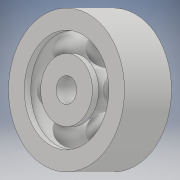
# Autodesk Inventor part: Подшипник
Saved by Autodesk Inventor 2018.1 (Build 221171000, 171)
## iProperties
Part Number: Подшипник
Material: Типовые
Document SubType Name: Modeling
Designer: User
Density: 1 g/cm^3
Appearance: По умолчанию
Author: User
Autodesk Inventor part; units mm, degrees
ref_plane "YZ Plane" through (0, 0, 0) normal (1, 0, 0) x (0, 1, 0)
ref_plane "XZ Plane" through (0, 0, 0) normal (0, 1, 0) x (-1, 0, 0)
ref_plane "XY Plane" through (0, 0, 0) normal (0, 0, 1) x (1, 0, 0)
sketch "Эскиз1" plane through (0, 0, 0) normal (0, 0, 1) x (1, 0, 0)
  line L0 (-3.5599, 1.7864) -> (-5.0501, 1.7864)
  line L1 (-5.0501, 1.7864) -> (-5.0501, 5.1167)
  line L2 (-5.0501, 5.1167) -> (4.9499, 5.1167)
  line L3 (4.9499, 5.1167) -> (4.9499, 1.7864)
  line L4 (4.9499, 1.7864) -> (3.5599, 1.7864)
  line L5 (-3.5957, -1.7133) -> (-5.0501, -1.7133)
  line L6 (-5.0501, -1.7133) -> (-5.0501, -5.0436)
  line L7 (-5.0501, -5.0436) -> (4.9499, -5.0436)
  line L8 (4.9499, -5.0436) -> (4.9499, -1.7133)
  line L9 (4.9499, -1.7133) -> (3.5957, -1.7133)
  arc A0 (-3.5957, -1.7133) -> (3.5957, -1.7133) centre (0, 0) ccw
  arc A1 (3.5599, 1.7864) -> (-3.5599, 1.7864) centre (0, 0) ccw
  line L10 (-5.0501, -7.2244) -> (4.9499, -7.2244)
  dimension "d6" = 10
  constraints: 22 end point, 6 perpendicular, 4 point on circle, 4 point on line, 3 horizontal, 2 centre point, 1 coincident, 1 collinear
  measures "d6" distance of L1.end L2.end
revolve "Вращение1" add sketch "Эскиз1" angle 360 about axis through (-5.0501, -7.2244, 0) along (1, 0, 0)
sketch "Эскиз2" plane through (0, 0, 0) normal (0, 0, 1) x (1, 0, 0)
  line L0 (0, 2.315) -> (0, -2.685)
  arc A0 (0, 2.315) -> (0, -2.685) centre (-0.5806, -0.185) ccw
  point P0 (0, 0)
  dimension "d7" = 5
  constraints: 2 end point, 2 point on circle, 1 centre point, 1 vertical
  measures "d7" distance of L0.start L0.end
revolve "Вращение2" add sketch "Эскиз2" angle 360 about axis through (0, 2.315, 0) along (0, -1, 0)
pattern_circular "Круговой массив1" count 6 over 360 about axis through (4.2549, -7.2244, 0) along (1, 0, 0) of "Вращение2"
